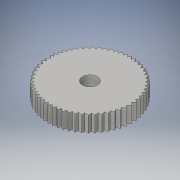
# Autodesk Inventor part: Part3
Saved by Autodesk Inventor 2016 (Build 200138000, 138)
## iProperties
Created: 2016-11-13
Part Number: Part3
Material: Generic
Document SubType Name: Modeling
Designer: adam fishburn
Density: 1 g/cm^3
Appearance: Default
Author: adam fishburn
Autodesk Inventor part; units mm, degrees
ref_plane "YZ Plane" through (0, 0, 0) normal (1, 0, 0) x (0, 1, 0)
ref_plane "XZ Plane" through (0, 0, 0) normal (0, 1, 0) x (-1, 0, 0)
ref_plane "XY Plane" through (0, 0, 0) normal (0, 0, 1) x (1, 0, 0)
sketch "Sketch1" plane through (0, 0, 0) normal (0, 1, 0) x (-1, 0, 0)
  line L0 (0, 0) -> (50.8, 0)
  line L1 (50.8, 0) -> (50.8, -50.8)
  line L2 (50.8, -50.8) -> (0, -50.8)
  line L3 (0, -50.8) -> (0, 0)
  dimension "d0" = 50.8
  dimension "d1" = 50.8
  constraints: 8 end point, 2 parallel, 1 horizontal, 1 perpendicular
  measures "d0" distance of L1.end L2.end
  measures "d1" distance of L0.end L1.end
extrude "Extrusion1" add sketch "Sketch1" along normal blind 6.35
sketch "Sketch2" plane through (0, 6.35, 0) normal (0, 1, 0) x (1, 0, 0)
  line L0 (-50.8, 0) -> (0, 0) projected
  line L1 (0, 50.8) -> (-50.8, 50.8) projected
  line L2 (0, 0) -> (0, 50.8) projected
  line L3 (-50.8, 50.8) -> (-50.8, 0) projected
  line L4 (-41.275, 25.4) -> (-42.3161, 26.3017)
  line L5 (-42.3161, 26.3017) -> (-41.2152, 26.7765)
  line L6 (-41.2152, 26.7765) -> (-42.1935, 27.6239)
  line L7 (-42.1935, 27.6239) -> (-41.0338, 28.1567)
  line L8 (-41.0338, 28.1567) -> (-41.9265, 29.1205)
  line L9 (-41.9265, 29.1205) -> (-40.7053, 29.6148)
  line L10 (-40.2288, 31.0677) -> (-40.8574, 32.3306)
  line L11 (-40.8574, 32.3306) -> (-39.6453, 32.4062)
  line L12 (-40.7053, 29.6148) -> (-41.5075, 30.6454)
  line L13 (-41.5075, 30.6454) -> (-40.2288, 31.0677)
  line L14 (-39.6453, 32.4062) -> (-40.1355, 33.7565)
  line L15 (-40.1355, 33.7565) -> (-38.8976, 33.7565)
  line L16 (-38.8976, 33.7565) -> (-39.2387, 35.1702)
  line L17 (-39.2387, 35.1702) -> (-37.9124, 35.1702)
  line L18 (-37.9124, 35.1702) -> (-38.0877, 36.6244)
  line L19 (-38.0877, 36.6244) -> (-36.7241, 36.5257)
  line L20 (-36.7241, 36.5257) -> (-36.811, 37.9202)
  line L21 (-36.811, 37.9202) -> (-35.3758, 37.7491)
  line L22 (-35.3758, 37.7491) -> (-35.2732, 39.1654)
  line L23 (-35.2732, 39.1654) -> (-33.8869, 38.816)
  line L24 (-33.8869, 38.816) -> (-33.6893, 40.1734)
  line L25 (-33.6893, 40.1734) -> (-32.4107, 39.6431)
  line L26 (-32.4107, 39.6431) -> (-32.0523, 40.9792)
  line L27 (-32.0523, 40.9792) -> (-30.7131, 40.3595)
  line L28 (-30.7131, 40.3595) -> (-30.4475, 41.5706)
  line L29 (-30.4475, 41.5706) -> (-29.3678, 40.7712)
  line L30 (-29.3678, 40.7712) -> (-28.7917, 41.9971)
  line L31 (-28.7917, 41.9971) -> (-27.6772, 41.1108)
  line L32 (-27.6772, 41.1108) -> (-27.0695, 42.2576)
  line L33 (-27.0695, 42.2576) -> (-26.1433, 41.2576)
  line L34 (-26.1433, 41.2576) -> (-25.4282, 42.34)
  line L35 (-25.4282, 42.34) -> (-24.7123, 41.2601)
  line L36 (-24.7123, 41.2601) -> (-23.906, 42.2741)
  line L37 (-23.906, 42.2741) -> (-23.2101, 41.1232)
  line L38 (-23.2101, 41.1232) -> (-22.2212, 42.0391)
  line L39 (-22.2212, 42.0391) -> (-21.5767, 40.8077)
  line L40 (-21.5767, 40.8077) -> (-20.368, 41.5754)
  line L41 (-20.368, 41.5754) -> (-19.836, 40.268)
  line L42 (-19.836, 40.268) -> (-18.5657, 40.9002)
  line L43 (-18.5657, 40.9002) -> (-18.2046, 39.5507)
  line L44 (-18.2046, 39.5507) -> (-16.9937, 40.1071)
  line L45 (-16.9937, 40.1071) -> (-16.7004, 38.679)
  line L46 (-16.7004, 38.679) -> (-15.3174, 39.0128)
  line L47 (-15.3174, 39.0128) -> (-15.1924, 37.5582)
  line L48 (-15.1924, 37.5582) -> (-13.7961, 37.7416)
  line L49 (-13.7961, 37.7416) -> (-13.866, 36.308)
  line L50 (-13.866, 36.308) -> (-12.4193, 36.2842)
  line L51 (-12.4193, 36.2842) -> (-12.6609, 34.8727)
  line L52 (-12.6609, 34.8727) -> (-11.2854, 34.7679)
  line L53 (-11.2854, 34.7679) -> (-11.6477, 33.3303)
  line L54 (-11.6477, 33.3303) -> (-10.2494, 32.9779)
  line L55 (-10.2494, 32.9779) -> (-10.7869, 31.6026)
  line L56 (-10.7869, 31.6026) -> (-9.5138, 31.2818)
  line L57 (-9.5138, 31.2818) -> (-10.1977, 29.9721)
  line L58 (-10.1977, 29.9721) -> (-8.9156, 29.3027)
  line L59 (-8.9156, 29.3027) -> (-9.7773, 28.2191)
  line L60 (-9.7773, 28.2191) -> (-8.5797, 27.4109)
  line L61 (-8.5797, 27.4109) -> (-9.55, 26.2907)
  line L62 (-9.55, 26.2907) -> (-8.4602, 25.296)
  line L63 (-8.4602, 25.296) -> (-9.5657, 24.264)
  line L64 (-9.5657, 24.264) -> (-8.5942, 23.2714)
  line L65 (-8.5942, 23.2714) -> (-9.8106, 22.4024)
  line L66 (-9.8106, 22.4024) -> (-8.9609, 21.3108)
  line L67 (-8.9609, 21.3108) -> (-10.2579, 20.632)
  line L68 (-10.2579, 20.632) -> (-9.5051, 19.5419)
  line L69 (-9.5051, 19.5419) -> (-10.8599, 19.028)
  line L70 (-10.8599, 19.028) -> (-10.2788, 17.7635)
  line L71 (-10.2788, 17.7635) -> (-11.6817, 17.4111)
  line L72 (-11.6817, 17.4111) -> (-11.2461, 16.0923)
  line L73 (-11.2461, 16.0923) -> (-12.6655, 15.9211)
  line L74 (-12.6655, 15.9211) -> (-12.4865, 14.4361)
  line L75 (-12.4865, 14.4361) -> (-13.8289, 14.5314)
  line L76 (-13.8289, 14.5314) -> (-13.762, 13.0905)
  line L77 (-13.762, 13.0905) -> (-15.245, 13.1979)
  line L78 (-15.245, 13.1979) -> (-15.2811, 11.8142)
  line L79 (-15.2811, 11.8142) -> (-16.6914, 12.1269)
  line L80 (-16.6914, 12.1269) -> (-16.8435, 10.7797)
  line L81 (-16.8435, 10.7797) -> (-18.3013, 11.2006)
  line L82 (-18.3013, 11.2006) -> (-18.563, 9.9009)
  line L83 (-18.563, 9.9009) -> (-19.788, 10.5501)
  line L84 (-19.788, 10.5501) -> (-20.2552, 9.2601)
  line L85 (-20.2552, 9.2601) -> (-21.5283, 10.0044)
  line L86 (-21.5283, 10.0044) -> (-22.0283, 8.7989)
  line L87 (-22.0283, 8.7989) -> (-23.0856, 9.6946)
  line L88 (-23.0856, 9.6946) -> (-23.8044, 8.5352)
  line L89 (-23.8044, 8.5352) -> (-24.6809, 9.5413)
  line L90 (-24.6809, 9.5413) -> (-25.3953, 8.4599)
  line L91 (-25.3953, 8.4599) -> (-26.263, 9.5485)
  line L92 (-26.263, 9.5485) -> (-27.1113, 8.5466)
  line L93 (-27.1113, 8.5466) -> (-27.8147, 9.7097)
  line L94 (-27.8147, 9.7097) -> (-28.7883, 8.8022)
  line L95 (-28.7883, 8.8022) -> (-29.2954, 10.0103)
  line L96 (-29.2954, 10.0103) -> (-30.3448, 9.1977)
  line L97 (-30.3448, 9.1977) -> (-30.7397, 10.45)
  line L98 (-30.7397, 10.45) -> (-31.8694, 9.7439)
  line L99 (-31.8694, 9.7439) -> (-32.1323, 11.0232)
  line L100 (-32.1323, 11.0232) -> (-33.5086, 10.5266)
  line L101 (-33.5086, 10.5266) -> (-33.6433, 11.833)
  line L102 (-33.6433, 11.833) -> (-35.0263, 11.4609)
  line L103 (-35.0263, 11.4609) -> (-35.0045, 12.76)
  line L104 (-35.0045, 12.76) -> (-36.3438, 12.4695)
  line L105 (-36.3438, 12.4695) -> (-36.2776, 13.8375)
  line L106 (-36.2776, 13.8375) -> (-37.7655, 13.8216)
  line L107 (-37.7655, 13.8216) -> (-37.5059, 15.1305)
  line L108 (-37.5059, 15.1305) -> (-38.9514, 15.2351)
  line L109 (-38.9514, 15.2351) -> (-38.7277, 16.7752)
  line L110 (-38.7277, 16.7752) -> (-40.1169, 17.0109)
  line L111 (-40.1169, 17.0109) -> (-39.6609, 18.4257)
  line L112 (-39.6609, 18.4257) -> (-41.0296, 18.8668)
  line L113 (-41.0296, 18.8668) -> (-40.3622, 20.0946)
  line L114 (-40.3622, 20.0946) -> (-41.646, 20.6006)
  line L115 (-41.646, 20.6006) -> (-40.8927, 21.9371)
  line L116 (-40.8927, 21.9371) -> (-42.1097, 22.6158)
  line L117 (-42.1097, 22.6158) -> (-41.1843, 23.7054)
  line L118 (-41.1843, 23.7054) -> (-42.3135, 24.4514)
  line L119 (-42.3135, 24.4514) -> (-41.275, 25.4)
  constraints: 232 end point, 3 perpendicular, 2 horizontal
extrude "Extrusion2" cut sketch "Sketch2" against normal blind 25.4
sketch "Sketch3" plane through (0, 6.35, 0) normal (0, 1, 0) x (1, 0, 0)
  line L0 (-41.1843, 23.7054) -> (-42.1097, 22.6158) projected
  line L1 (-9.5138, 31.2818) -> (-10.7869, 31.6026) projected
  line L2 (-38.0877, 36.6244) -> (-37.9124, 35.1702) projected
  line L3 (-18.5657, 40.9002) -> (-19.836, 40.268) projected
  line L4 (-33.6433, 11.833) -> (-33.5086, 10.5266) projected
  line L5 (-42.3161, 26.3017) -> (-41.275, 25.4) projected
  circle A0 centre (-25.4, 25.4) radius 3
  point P0 (0, 0)
  point P1 (-8.4602, 25.296)
  dimension "d9" = 6
  constraints: 1 centre point
  measures "d9" diameter of A0
extrude "Extrusion3" cut sketch "Sketch3" against normal blind 6.35
body "Solid1"
